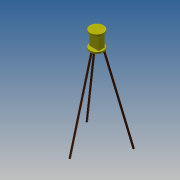
# Autodesk Inventor part: totalStation
Saved by Autodesk Inventor 2014 SP1 (Build 180222100, 222)
## iProperties
Created: 2014-08-28
Part Number: totalStation
Material: Generic
Document SubType Name: Modeling
Designer: Dave
Density: 1 g/cm^3
Appearance: Default
Author: Dave
Autodesk Inventor part; units mm, degrees
ref_plane "YZ Plane" through (0, 0, 0) normal (1, 0, 0) x (0, 1, 0)
ref_plane "XZ Plane" through (0, 0, 0) normal (0, 1, 0) x (-1, 0, 0)
sketch "Sketch1" plane through (0, 0, 0) normal (0, 1, 0) x (-1, 0, 0)
  circle A0 centre (0, 0) radius 101.6
  dimension "d0" = 203.2
  constraints: 1 centre point, 1 coincident
  measures "d0" diameter of A0
extrude "Extrusion1" add sketch "Sketch1" along normal blind 25.4
sketch "Sketch2" plane through (0, 0, 0) normal (0, -1, 0) x (1, 0, 0)
  circle A0 centre (0, 0) radius 101.6 projected
  point P0 (0, 101.6)
  constraints: 1 vertical alignment, 1 other
ref_plane "Work Plane1" through (0, 0, 101.6) normal (0, 0, 1) x (1, 0, 0)
sketch "Sketch3" plane through (0, 0, 101.6) normal (0, 0, 1) x (1, 0, 0)
  line L0 (0, 0) -> (50.8, 0) construction
  dimension "d3" = 50.8
  constraints: 2 end point, 1 horizontal
  measures "d3" distance of L0.start L0.end
ref_plane "Work Plane2" through (0, 0, 101.6) normal (0, -0.9659, 0.2588) x (1, 0, 0)
sketch "Sketch4" plane through (0, 0, 101.6) normal (0, -0.9659, 0.2588) x (1, 0, 0)
  line L0 (-19.0468, -4.4588) -> (19.0532, -4.4588)
  line L1 (19.0532, -4.4588) -> (19.0532, -42.5588)
  line L2 (19.0532, -42.5588) -> (-19.0468, -42.5588)
  line L3 (-19.0468, -42.5588) -> (-19.0468, -4.4588)
  point P0 (0, -98.1381)
  point P1 (0.0032, -0.0121)
  dimension "d5" = 38.1
  dimension "d6" = 38.1
  constraints: 8 end point, 2 parallel, 1 horizontal, 1 perpendicular
  measures "d5" distance of L1.end L2.end
  measures "d6" distance of L2.end L0.start
extrude "Extrusion2" add sketch "Sketch4" against normal blind 25.4
sketch "Sketch5" plane through (0, 0, 101.6) normal (0, -0.9659, 0.2588) x (1, 0, 0)
  circle A0 centre (0, -23.5088) radius 12.7
  point P0 (0, -98.1381)
  dimension "d9" = 25.4
  constraints: 1 centre point
  measures "d9" diameter of A0
extrude "Extrusion3" add sketch "Sketch5" along normal blind 1270
pattern_circular "Circular Pattern2" count 3 over 360 about axis through (0, 0, 0) along (0, 1, 0) of "Extrusion2", "Extrusion3"
sketch "Sketch6" plane through (0, 25.4, 0) normal (0, 1, 0) x (1, 0, 0)
  line L0 (-68.8618, -43.3163) -> (73.3045, -43.3163)
  line L1 (73.3045, -43.3163) -> (73.3045, 47.759)
  line L2 (73.3045, 47.759) -> (-68.8618, 47.759)
  line L3 (-68.8618, 47.759) -> (-68.8618, -43.3163)
  constraints: 8 end point, 2 parallel, 1 horizontal, 1 perpendicular
extrude "Extrusion4" add sketch "Sketch6" along normal blind 203.2
sketch "Sketch8" plane through (0, 228.6, 0) normal (0, 1, 0) x (1, 0, 0)
  circle A0 centre (0, 0) radius 101.6
  dimension "d23" = 203.2
  constraints: 1 centre point, 1 coincident
  measures "d23" diameter of A0
extrude "Extrusion6" add sketch "Sketch8" along normal blind 25.4
body "Solid1"
